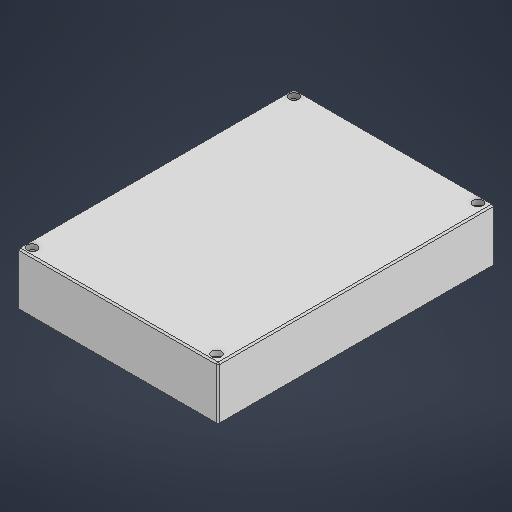
# Autodesk Inventor part: Kameraturm_Deckel
Saved by Autodesk Inventor 2026.1 (Build 301233020, 233B)
## iProperties
Created: 2025-08-17
Part Number: Kameraturm_Deckel
Material: Generic
Document SubType Name: Modeling
Designer: peter
Density: 1 g/cm^3
Appearance: Default
Author: peter
Autodesk Inventor part; units mm, degrees
ref_plane "YZ Plane" through (0, 0, 0) normal (1, 0, 0) x (0, 1, 0)
ref_plane "XZ Plane" through (0, 0, 0) normal (0, 1, 0) x (-1, 0, 0)
ref_plane "XY Plane" through (0, 0, 0) normal (0, 0, 1) x (1, 0, 0)
sketch "Sketch1" plane through (0, 0, 0) normal (0, 0, 1) x (1, 0, 0)
  line L0 (-61.5, -83.5) -> (62.5, -83.5)
  line L1 (62.5, -83.5) -> (62.5, 73.5)
  line L2 (62.5, 73.5) -> (-61.5, 73.5)
  line L3 (-61.5, 73.5) -> (-61.5, -83.5)
  line L4 (-67.5, -94.5) -> (67.5, -94.5) projected
  line L5 (67.5, -94.5) -> (67.5, 91.5) projected
  line L6 (62.5, -70.5) -> (-20.5, -70.5) projected
  line L7 (-20.5, 73.5) -> (62.5, 73.5) projected
  line L8 (62.5, 73.5) -> (62.5, -70.5) projected
  line L9 (67.5, 91.5) -> (-67.5, 91.5) projected
  line L10 (-67.5, 91.5) -> (-67.5, -94.5) projected
  circle A0 centre (61.2932, 86.5) radius 2 projected
  circle A1 centre (61.2932, -89.3536) radius 2 projected
  circle A2 centre (-62.5, -89.3536) radius 2 projected
  circle A3 centre (-62.5, 86.5) radius 2 projected
  line L11 (-64.5, -83.5) -> (-64.5, 80.5) projected
  line L12 (-58.5, 86.5) -> (-64.5, 80.5) projected
  line L13 (-58.5, 86.5) -> (-30.5, 86.5) projected
  line L14 (-30.5, 86.5) -> (-30.5, 24) projected
  line L15 (-30.5, 24) -> (-20.5, 24) projected
  line L16 (-20.5, 24) -> (-20.5, 73.5) projected
  line L17 (-20.5, -70.5) -> (-20.5, -21) projected
  line L18 (-20.5, -21) -> (-30.5, -21) projected
  line L19 (-30.5, -21) -> (-30.5, -89.5) projected
  line L20 (-30.5, -89.5) -> (-58.5, -89.5) projected
  line L21 (-64.5, -83.5) -> (-58.5, -89.5) projected
  point P0 (0, 0)
  point P1 (67.5, -91)
  point P2 (67, 91.5)
  point P3 (-67, 91.5)
  point P4 (-67.5, 91)
  constraints: 8 end point, 2 parallel, 1 horizontal, 1 perpendicular
extrude "Extrusion1" add sketch "Sketch1" along normal blind 35 contours L3 L2 L14 L15 L16 L1 L6 L17 L18 L19 L0 | L0 L19 L20 L21 L11 L12 L13 L14 L2 L3 | L19 L18 L17 L6 L1 L0 | L2 L16 L15 L14 | L10 L9 L5 L4 | A0 | A1 | A2 | A3
sketch "Skizze3" plane through (0, 0, 35) normal (0, 0, 1) x (1, 0, 0)
  circle A0 centre (61.2932, 86.5) radius 2 projected
  circle A1 centre (-62.5, 86.5) radius 2 projected
  circle A2 centre (61.2932, -89.3536) radius 2 projected
  circle A3 centre (-62.5, -89.3536) radius 2 projected
  point P0 (0, 0)
hole "Bohrung1" at (-62.5, 86.5, 35) at (61.2932, 86.5, 35) at (61.2932, -89.3536, 35) at (-62.5, -89.3536, 35) direction (0, 0, -1) diameter 3.4 end through all counterbore diameter 6.5 counterbore depth 3.4 clearance for "Inbusschraube DIN EN ISO 4762" size "M3" standard "DIN"
sketch "Skizze4" plane through (0, 0, 0) normal (0, 0, -1) x (-1, 0, 0)
  line L0 (-57.5, 84.5) -> (57.5, 84.5)
  line L1 (57.5, 84.5) -> (57.5, -84.5)
  line L2 (57.5, -84.5) -> (-57.5, -84.5)
  line L3 (-57.5, -84.5) -> (-57.5, 84.5)
  line L4 (-57.5, 84.5) -> (57.5, -84.5) construction
  line L5 (57.5, 84.5) -> (-57.5, -84.5) construction
  line L6 (67.5, 91.5) -> (67.5, -94.5) projected
  line L7 (67.5, -94.5) -> (-67.5, -94.5) projected
  point P0 (0, 0)
  dimension "d14" = 10
  dimension "d15" = 10
  constraints: 12 end point, 2 midpoint, 2 parallel, 1 horizontal, 1 perpendicular
  measures "d14" distance between parallel lines of L6 L1
  measures "d15" distance between parallel lines of L7 L2
extrude "Extrusion3" cut sketch "Skizze4" against normal blind 30
chamfer "Fasen2" distance 1 angle 45 4 edges at (-67.5, -94.5, 17.5) (-67.5, 91.5, 17.5) (67.5, 91.5, 17.5) (67.5, -94.5, 17.5)
chamfer "Fasen3" distance 1 angle 45 8 edges at (-67.5, -1.5, 35) (0, 91.5, 35) (67.5, -1.5, 35) (0, -94.5, 35) (-67, -94, 35) (67, -94, 35) (67, 91, 35) (-67, 91, 35)
body "Solid1"
